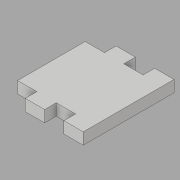
# Autodesk Inventor part: e
Saved by Autodesk Inventor 2019 (Build 230136000, 136)
## iProperties
Created: 2021-11-01
Part Number: e
Material: Generic
Document SubType Name: Modeling
Designer: Mohamed
Density: 1 g/cm^3
Appearance: Default
Author: Mohamed
Autodesk Inventor part; units mm, degrees
ref_plane "YZ Plane" through (0, 0, 0) normal (1, 0, 0) x (0, 1, 0)
ref_plane "XZ Plane" through (0, 0, 0) normal (0, 1, 0) x (-1, 0, 0)
ref_plane "XY Plane" through (0, 0, 0) normal (0, 0, 1) x (1, 0, 0)
sketch "Sketch1" plane through (0, 0, 0) normal (0, 1, 0) x (-1, 0, 0)
  line L0 (0, 0) -> (40, 0)
  line L1 (40, 0) -> (40, -35)
  line L2 (40, -35) -> (0, -35)
  line L3 (0, -35) -> (0, 0)
  dimension "d0" = 40
  dimension "d1" = 35
  constraints: 8 end point, 2 parallel, 1 horizontal, 1 perpendicular
  measures "d0" distance of L1.end L2.end
  measures "d1" distance of L0.end L1.end
extrude "Extrusion1" add sketch "Sketch1" along normal blind 6
sketch "Sketch2" plane through (0, 6, 0) normal (0, 1, 0) x (1, 0, 0)
  line L0 (-40, 35) -> (-40, 0) projected
  line L1 (-40, 0) -> (-30, 0)
  line L2 (-40, 0) -> (0, 0) projected
  line L3 (-30, 0) -> (-20, 0)
  line L4 (-20, 0) -> (-20, -6)
  line L5 (-20, -6) -> (-30, -6)
  line L6 (-30, -6) -> (-30, 0)
  line L7 (-30, 35) -> (-20, 35)
  line L8 (-20, 35) -> (-20, 41)
  line L9 (-20, 41) -> (-30, 41)
  line L10 (-30, 41) -> (-30, 35)
  dimension "d4" = 10
  dimension "d5" = 10
  dimension "d6" = 6
  dimension "d7" = 10
  dimension "d8" = 6
  constraints: 18 end point, 4 parallel, 2 horizontal, 2 perpendicular, 1 point on line
  measures "d4" distance of L0.end L1.end
  measures "d5" distance of L4.end L5.end
  measures "d6" distance of L3.end L4.end
  measures "d7" distance of L9.end L8.end
  measures "d8" distance of L8.end L7.end
extrude "Extrusion2" add sketch "Sketch2" against normal blind 6
pattern_linear "Rectangular Pattern1" count 2 spacing 20 along (1, 0, 0) of "Extrusion2"
body "Solid1"
